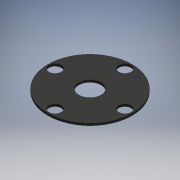
# Autodesk Inventor part: Black Rubber Pad Bottom
Saved by Autodesk Inventor 2017 (Build 210142000, 142)
## iProperties
Created: 2020-05-28
Part Number: Black Rubber Pad Bottom
Material: Generic
Document SubType Name: Modeling
Designer: Sid
Density: 1 g/cm^3
Appearance: Default
Author: Sid
Autodesk Inventor part; units mm, degrees
ref_plane "YZ Plane" through (0, 0, 0) normal (1, 0, 0) x (0, 1, 0)
ref_plane "XZ Plane" through (0, 0, 0) normal (0, 1, 0) x (-1, 0, 0)
ref_plane "XY Plane" through (0, 0, 0) normal (0, 0, 1) x (1, 0, 0)
sketch "Sketch1" plane through (0, 0, 0) normal (0, 0, 1) x (1, 0, 0)
  circle A0 centre (0, 0) radius 34
  circle A1 centre (0, 0) radius 9
  circle A2 centre (0, 28.25) radius 5
  circle A3 centre (-28.25, 0) radius 5
  circle A4 centre (0, -28.25) radius 5
  circle A5 centre (28.25, 0) radius 5
  arc A6 (4.9804, 27.8075) -> (-4.9804, 27.8075) centre (0, 0) ccw
  arc A7 (27.8075, -4.9804) -> (27.8075, 4.9804) centre (0, 0) ccw
  arc A8 (-27.8075, 4.9804) -> (-27.8075, -4.9804) centre (0, 0) ccw
  arc A9 (-4.9804, -27.8075) -> (4.9804, -27.8075) centre (0, 0) ccw
  dimension "d0" = 68
  dimension "d1" = 18
  dimension "d3" = 10
  dimension "d6" = 360
  constraints: 17 point on circle, 10 centre point, 3 coincident, 9 other
  measures "d0" diameter of A0
  measures "d1" diameter of A1
  measures "d3" diameter of A2
extrude "Extrusion1" add sketch "Sketch1" along normal blind 2
body "Solid1"
